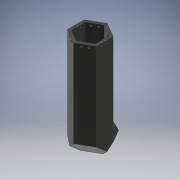
# Autodesk Inventor part: A01
Saved by Autodesk Inventor 2017 (Build 210142000, 142)
## iProperties
Created: 2019-09-19
Part Number: A01
Material: ABS Plastic
Document SubType Name: Modeling
Designer: Dell
Density: 1.06 g/cm^3
Appearance: Smooth - Black
Mass: 2688.13 g
Surface Area: 1514.93 cm^2
Volume: 2535.97 cm^3
Author: Dell
Autodesk Inventor part; units mm, degrees
ref_plane "YZ Plane" through (0, 0, 0) normal (1, 0, 0) x (0, 1, 0)
ref_plane "XZ Plane" through (0, 0, 0) normal (0, 1, 0) x (-1, 0, 0)
ref_plane "XY Plane" through (0, 0, 0) normal (0, 0, 1) x (1, 0, 0)
sketch "Sketch1" plane through (0, 0, 0) normal (0, 0, 1) x (1, 0, 0)
  line L0 (0, 46.188) -> (40, 23.094)
  line L1 (40, 23.094) -> (40, -23.094)
  line L2 (40, -23.094) -> (0, -46.188)
  line L3 (0, -46.188) -> (-40, -23.094)
  line L4 (-40, -23.094) -> (-40, 23.094)
  line L5 (-40, 23.094) -> (0, 46.188)
  line L6 (0, 38.1051) -> (33, 19.0526)
  line L7 (33, 19.0526) -> (33, -19.0526)
  line L8 (33, -19.0526) -> (0, -38.1051)
  line L9 (0, -38.1051) -> (-33, -19.0526)
  line L10 (-33, -19.0526) -> (-33, 19.0526)
  line L11 (-33, 19.0526) -> (0, 38.1051)
  point P0 (0, 0)
  point P1 (0, 0)
  dimension "d1" = 66
  dimension "d45" = 7
  constraints: 24 end point, 1 coincident, 1 vertical alignment, 18 other
  measures "d1" distance between parallel lines of L7 L10
  measures "d45" distance between parallel lines of L1 L7
extrude "Extrusion1" add sketch "Sketch1" along normal blind 250
sketch "Sketch2" plane through (40, -23.094, 0) normal (1, 0, 0) x (0, 0, -1)
  line L0 (-243.5, 15.594) -> (-243.5, 30.594) construction
  line L1 (-250, 0) -> (-250, 46.188) projected
  circle A0 centre (-243.5, 30.594) radius 2.5
  circle A1 centre (-243.5, 15.594) radius 2.5
  point P0 (0, 23.094)
  point P1 (-243.5, 23.094)
  point P2 (-250, 23.094)
  dimension "d4" = 15
  dimension "d5" = 6.5
  dimension "d6" = 5
  dimension "d7" = 5
  constraints: 2 centre point, 2 coincident, 2 end point, 2 midpoint, 1 horizontal alignment, 1 vertical
  measures "d4" distance of L0.start L0.end
  measures "d5" distance between parallel lines of L0 L1
  measures "d6" diameter of A0
  measures "d7" diameter of A1
extrude "Extrusion2" cut sketch "Sketch2" against normal blind 30
pattern_circular "Circular Pattern1" count 6 over 360 about axis through (0, 0, -10) along (0, 0, 1) of "Extrusion2"
sketch "Sketch8" plane through (-40, 23.094, 250) normal (-0.5, 0.8660254, 0) x (0.8660254, 0.5, 0)
  line L0 (42.1466, 250) -> (4.0415, 250) projected
  line L1 (-23.094, 250) -> (0, 250) projected
  line L2 (-23.094, 250) -> (0, 290)
  line L3 (0, 290) -> (46.188, 290)
  line L4 (46.188, 290) -> (69.282, 250)
  line L5 (69.282, 250) -> (46.188, 210)
  line L6 (46.188, 210) -> (0, 210)
  line L7 (0, 210) -> (-23.094, 250)
  point P0 (23.094, 250)
  constraints: 12 end point, 1 midpoint, 13 other
extrude "Extrusion6" add sketch "Sketch8" against normal up to surface (80 mm away) from surface at 0
sketch "Sketch9" plane through (0, 0, 250) normal (0, 0, 1) x (1, 0, 0)
  line L0 (-40, -23.094) -> (0, -46.188) projected
  line L1 (-20, -57.735) -> (-40, -23.094) projected
  line L2 (-20, -57.735) -> (0, -46.188) projected
  line L3 (40, -23.094) -> (40, 23.094) projected
  line L4 (40, -23.094) -> (60, -11.547) projected
  line L5 (40, 23.094) -> (60, -11.547) projected
  point P0 (0, 0)
extrude "Extrusion7" cut sketch "Sketch9" against normal through all
sketch "Sketch10" plane through (-40, 23.094, 250) normal (-0.5, 0.8660254, 0) x (0.8660254, 0.5, 0)
  line L0 (-13.8564, 250) -> (4.6188, 282)
  line L1 (4.6188, 282) -> (41.5692, 282)
  line L2 (41.5692, 282) -> (60.0444, 250)
  line L3 (60.0444, 250) -> (41.5692, 218)
  line L4 (41.5692, 218) -> (4.6188, 218)
  line L5 (4.6188, 218) -> (-13.8564, 250)
  line L6 (0, 290) -> (46.188, 290) projected
  point P0 (23.094, 250)
  point P1 (23.094, 250)
  point P2 (23.094, 282)
  point P3 (23.094, 290)
  dimension "d32" = 64
  constraints: 12 end point, 2 midpoint, 1 coincident, 1 vertical alignment, 13 other
  measures "d32" distance between parallel lines of L1 L4
extrude "Extrusion8" add sketch "Sketch10" along normal blind 13
sketch "Sketch11" plane through (-46.5, 34.3523, 250) normal (-0.5, 0.8660254, 0) x (0.8660254, 0.5, 0)
  circle A0 centre (23.094, 250) radius 12.5
  dimension "d35" = 25
  constraints: 1 centre point, 1 coincident
  measures "d35" diameter of A0
extrude "Extrusion9" cut sketch "Sketch11" against normal blind 69.5
sketch "Sketch13" plane through (-33, 10.9697, 40) normal (0, 0, 1) x (1, 0, 0)
  line L0 (0, 0) -> (0, 8.0829) projected
  line L1 (0, 0) -> (26, -45.0333) projected
  line L2 (33, -49.0748) -> (26, -45.0333) projected
  line L3 (66, -30.0222) -> (33, -49.0748) projected
  line L4 (66, -21.9393) -> (66, -30.0222) projected
  line L5 (40, 23.094) -> (66, -21.9393) projected
  line L6 (33, 27.1355) -> (40, 23.094) projected
  line L7 (0, 8.0829) -> (33, 27.1355) projected
  line L8 (40, 23.094) -> (66, 8.0829) projected
  line L9 (40, 23.094) -> (66, -21.9393) projected
  line L10 (66, 8.0829) -> (66, -21.9393) projected
  line L11 (0, -30.0222) -> (0, 0) projected
  line L12 (26, -45.0333) -> (0, -30.0222) projected
  line L13 (0, 0) -> (26, -45.0333) projected
  point P0 (33, -10.9697)
extrude "Extrusion11" cut sketch "Sketch13" against normal blind 56.5
chamfer "Chamfer1" distance 50 angle 45 1 edges at (20, -34.641, -40)
sketch "Sketch14" plane through (15, 20.2073, -40) normal (0.3535534, -0.6123724, -0.7071068) x (-0.8660254, -0.5, 0)
  line L0 (-7.2169, -33.234) -> (53.4049, -33.234) projected
  line L1 (53.4049, -33.234) -> (42.1466, -60.8112) projected
  line L2 (42.1466, -60.8112) -> (4.0415, -60.8112) projected
  line L3 (4.0415, -60.8112) -> (-7.2169, -33.234) projected
  line L4 (60.6218, -35.3553) -> (46.188, 0) projected
  line L5 (46.188, 0) -> (0, 0) projected
  line L6 (0, 0) -> (-14.4338, -35.3553) projected
  line L7 (-14.4338, -35.3553) -> (0, -70.7107) projected
  line L8 (0, -70.7107) -> (46.188, -70.7107) projected
  line L9 (46.188, -70.7107) -> (60.6218, -35.3553) projected
  point P0 (23.094, -35.3553)
extrude "Extrusion12" add sketch "Sketch14" against normal blind 7 contours L0 L1 L2 L3 | L9 L8 L7 L6 L5 L4
sketch "Sketch15" plane through (20, 57.735, 0) normal (0.75, 0.4330127, -0.5) x (-0.4330127, -0.25, -0.8660254)
  line L0 (46.188, -30) -> (17.3205, -55) projected
  line L1 (46.188, 0) -> (46.188, -30) projected
  line L2 (46.188, 0) -> (0, 0) projected
  line L3 (0, 0) -> (0, -40) projected
  line L4 (0, -40) -> (17.3205, -55) projected
  line L5 (19.0526, -42.5) -> (16.1658, -40) projected
  line L6 (16.1658, -40) -> (19.0526, -37.5) projected
  line L7 (19.0526, -37.5) -> (19.0526, -42.5) projected
  point P0 (23.094, -40)
extrude "Extrusion13" add sketch "Sketch15" against normal blind 7 contours L0 L4 L3 L2 L1 | L5 L6 L7
sketch "Sketch16" plane through (-40, 23.094, -40) normal (-0.75, -0.4330127, -0.5) x (-0.4330127, -0.25, 0.8660254)
  line L0 (28.8675, -55) -> (0, -30) projected
  line L1 (28.8675, -55) -> (46.188, -40) projected
  line L2 (46.188, -40) -> (46.188, 0) projected
  line L3 (46.188, 0) -> (0, 0) projected
  line L4 (0, 0) -> (0, -30) projected
  line L5 (30.0222, -40) -> (27.1355, -42.5) projected
  line L6 (27.1355, -42.5) -> (27.1355, -37.5) projected
  line L7 (27.1355, -37.5) -> (30.0222, -40) projected
  point P0 (23.094, -40)
extrude "Extrusion14" add sketch "Sketch16" against normal blind 7 contours L0 L4 L3 L2 L1 | L5 L6 L7
body "Solid1"
